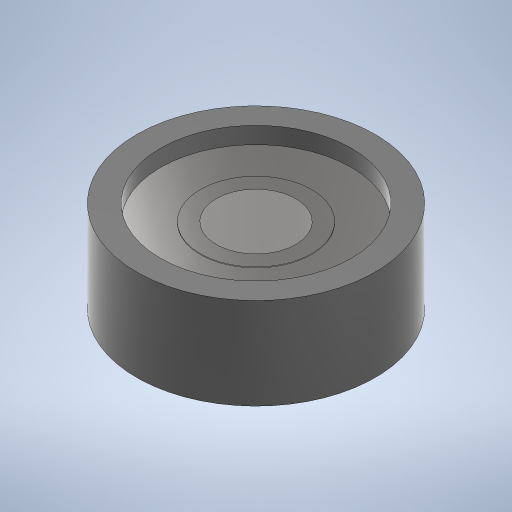
# Autodesk Inventor part: Gbear_30_10
Saved by Autodesk Inventor 2024.2 (Build 282272000, 272)
## iProperties
Created: 2024-03-24
Part Number: Gbear_30_10
Material: ステンレス鋼
Document SubType Name: Modeling
Designer: fhbdh
Density: 8 g/cm^3
Appearance: 半つや出し
Author: fhbdh
Autodesk Inventor part; units mm, degrees
ref_plane "YZ Plane" through (0, 0, 0) normal (1, 0, 0) x (0, 1, 0)
ref_plane "XZ Plane" through (0, 0, 0) normal (0, 1, 0) x (-1, 0, 0)
ref_plane "XY Plane" through (0, 0, 0) normal (0, 0, 1) x (1, 0, 0)
sketch "スケッチ1" plane through (0, 0, 0) normal (0, 0, 1) x (1, 0, 0)
  line L0 (-15, 5.75) -> (-15, -5.75)
  line L1 (-15, -5.75) -> (-12, -5.75)
  line L2 (-12, -5.75) -> (-12, -3.65)
  line L3 (-12, -3.65) -> (-7, -3.65)
  line L4 (-7, -3.65) -> (-7, -3.75)
  line L5 (-7, -3.75) -> (-5, -3.75)
  line L6 (-5, -3.75) -> (-5, 3.75)
  line L7 (0, 0) -> (-15, 0) construction
  line L8 (-15, 5.75) -> (-12, 5.75)
  line L9 (-12, 5.75) -> (-12, 3.65)
  line L10 (-12, 3.65) -> (-7, 3.65)
  line L11 (-7, 3.65) -> (-7, 3.75)
  line L12 (-7, 3.75) -> (-5, 3.75)
  line L13 (0, 0) -> (0, 5.75) construction
  point P0 (-5, 0)
  dimension "d0" = 11.5
  dimension "d1" = 15
  dimension "d2" = 5
  dimension "d3" = 0.1
  dimension "d4" = 2
  dimension "d5" = 3
  dimension "d6" = 2
  constraints: 28 end point, 6 perpendicular, 4 symmetric about line, 2 midpoint, 2 point on line, 2 vertical, 1 horizontal
  measures "d0" distance of L0.start L0.end
  measures "d1" distance from line of L7.start L0
  measures "d2" distance from line of L7.start L6
  measures "d3" distance between parallel lines of L3 L5
  measures "d4" distance between parallel lines of L5 L1
  measures "d5" distance of L0.end L1.end
  measures "d6" distance of L4.end L5.end
revolve "回転1" add sketch "スケッチ1" angle 360 about axis through (0, 0, 0) along (0, 1, 0)
